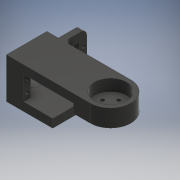
# Autodesk Inventor part: 第一臂-1
Saved by Autodesk Inventor 2017 (Build 210142000, 142)
## iProperties
Part Number: 第一臂-1
Material: 熱塑性塑膠樹脂
Document SubType Name: Modeling
Designer: Brian
Density: 1.28 g/cm^3
Appearance: 平滑 - 黑色
Mass: 49.9577 g
Surface Area: 163.253 cm^2
Volume: 39.0295 cm^3
Author: Brian
Autodesk Inventor part; units mm, degrees
ref_plane "YZ Plane" through (0, 0, 0) normal (1, 0, 0) x (0, 1, 0)
ref_plane "XZ Plane" through (0, 0, 0) normal (0, 1, 0) x (-1, 0, 0)
ref_plane "XY Plane" through (0, 0, 0) normal (0, 0, 1) x (1, 0, 0)
sketch "草圖1" plane through (0, 0, 0) normal (0, 0, 1) x (1, 0, 0)
  circle A0 centre (0, 0) radius 17.5
  circle A1 centre (120, 0) radius 17.5
  line L0 (0, 17.5) -> (120, 17.5)
  line L1 (120, 17.5) -> (120, -17.5)
  line L2 (120, -17.5) -> (0, -17.5)
  line L3 (0, -17.5) -> (0, 17.5)
  dimension "d0" = 35
  dimension "d1" = 35
  dimension "d4" = 120
  dimension "d5" = 35
  constraints: 8 end point, 3 coincident, 2 centre point, 2 midpoint, 2 parallel, 1 horizontal, 1 perpendicular
  measures "d0" diameter of A0
  measures "d1" diameter of A1
  measures "d4" distance of L0.start L0.end
  measures "d5" distance between parallel lines of L2 L0
extrude "擠出1" add sketch "草圖1" along normal blind 15
sketch "草圖2" plane through (0, 0, 15) normal (0, 0, 1) x (1, 0, 0)
  circle A0 centre (0, 0) radius 14
  arc A1 (120, -17.5) -> (120, 17.5) centre (120, 0) ccw projected
  circle A2 centre (120, 0) radius 14
  dimension "d6" = 28
  dimension "d7" = 28
  constraints: 2 centre point, 2 coincident
  measures "d6" diameter of A2
  measures "d7" diameter of A0
extrude "擠出2" cut sketch "草圖2" against normal blind 10
sketch "草圖5" plane through (0, 0, 0) normal (0, 0, -1) x (-1, 0, 0)
  circle A0 centre (0, 0) radius 14 projected
  line L0 (0, 17.5) -> (-120, 17.5) projected
  arc A1 (-120, 17.5) -> (-120, -17.5) centre (-120, 0) ccw projected
  line L1 (-120, -17.5) -> (0, -17.5) projected
  arc A2 (0, -17.5) -> (0, 17.5) centre (0, 0) ccw projected
  line L2 (0, 17.5) -> (-120, 17.5) projected
  line L3 (-87.5, 17.5) -> (-87.5, -17.5)
  line L4 (-120, -17.5) -> (0, -17.5) projected
  dimension "d13" = 50
  constraints: 2 end point, 2 point on line, 1 perpendicular
extrude "擠出4" add sketch "草圖5" along normal blind 20 contours A0 | A2 L1 L3 L0
ref_plane "工作平面1" through (0, 17.5, 11.7503) normal (0, 1, 0) x (1, 0, 0)
sketch "草圖6" plane through (0, 17.5, 11.7503) normal (0, 1, 0) x (1, 0, 0)
  line L0 (47.5, -10.5319) -> (-53.2917, -10.5319)
  line L1 (-53.2917, -10.5319) -> (-53.2917, 69.2461)
  line L2 (-53.2917, 69.2461) -> (47.5, 69.2461)
  line L3 (47.5, 69.2461) -> (47.5, -10.5319)
  line L4 (87.5, 11.7503) -> (87.5, 31.7503) projected
  point P0 (0, 11.7503)
  dimension "d19" = 40
  constraints: 8 end point, 2 parallel, 1 horizontal, 1 perpendicular
  measures "d19" distance between parallel lines of L4 L3
extrude "擠出5" cut sketch "草圖6" against normal through all
sketch "草圖7" plane through (120, 17.5, 15) normal (0, 1, 0) x (1, 0, 0)
  line L0 (-64.5, 7.25) -> (-14.5, 7.25)
  line L1 (-14.5, 7.25) -> (-14.5, 27.75)
  line L2 (-14.5, 27.75) -> (-64.5, 27.75)
  line L3 (-64.5, 27.75) -> (-64.5, 7.25)
  line L4 (0, 0) -> (-72.5, 0) projected
  line L5 (-72.5, 35) -> (-72.5, 0) projected
  point P0 (-120, 15)
  dimension "d20" = 20.5
  dimension "d21" = 7.25
  dimension "d22" = 8
  dimension "d23" = 50
  constraints: 8 end point, 2 parallel, 1 horizontal, 1 perpendicular
  measures "d20" distance of L2.end L0.start
  measures "d21" distance between parallel lines of L4 L0
  measures "d22" distance between parallel lines of L5 L3
  measures "d23" distance of L1.end L2.end
extrude "擠出6" cut sketch "草圖7" against normal through all
sketch "草圖8" plane through (47.5, -17.5, 15) normal (-1, 0, 0) x (0, 0, 1)
  line L0 (0, 0) -> (-35, 0) projected
  line L1 (0, 0) -> (-35, 35)
  line L2 (-35, 0) -> (-35, 35) projected
  circle A0 centre (-17.5, 17.5) radius 10.5
  point P0 (-15, 17.5)
  dimension "d26" = 21
  constraints: 2 end point, 1 centre point, 1 midpoint
  measures "d26" diameter of A0
extrude "擠出7" cut sketch "草圖8" against normal blind 10 contours A0 L1 | L1 A0
sketch "草圖9" plane through (120, 0, 5) normal (0, 0, 1) x (1, 0, 0)
  circle A0 centre (0, 0) radius 7
  circle A1 centre (0, 0) radius 14 projected
  line L0 (-7, 0) -> (0, 7)
  line L1 (0, 7) -> (7, 0)
  line L2 (7, 0) -> (0, -7)
  line L3 (0, -7) -> (-7, 0)
  point P0 (-120, 0)
  dimension "d29" = 14
  constraints: 8 end point, 1 coincident, 1 horizontal alignment, 12 other
hole "孔1" at (113, 0, 5) at (127, 0, 5) at (120, -7, 5) at (120, 7, 5) direction (0, 0, -1) diameter 3.2 depth 8 tip angle 118
sketch "草圖10" plane through (0, 0, 0) normal (0, 0, -1) x (-1, 0, 0)
  arc A0 (-120, 17.5) -> (-120, -17.5) centre (-120, 0) ccw projected
  circle A1 centre (-120, 0) radius 10
  circle A2 centre (-120, -7) radius 1.6 projected
  circle A3 centre (-113, 0) radius 1.6 projected
  circle A4 centre (-127, 0) radius 1.6 projected
  circle A5 centre (-120, 7) radius 1.6 projected
  line L0 (-105.5, -17.5) -> (-105.5, 17.5) projected
  line L1 (-105.5, 17.5) -> (-120, 17.5) projected
  arc A6 (-120, 17.5) -> (-120, -17.5) centre (-120, 0) ccw projected
  line L2 (-120, -17.5) -> (-105.5, -17.5) projected
  point P0 (0, 0)
  dimension "d37" = 20
  constraints: 1 centre point, 1 coincident
  measures "d37" diameter of A1
extrude "擠出8" add sketch "草圖10" along normal blind 0.2 contours A1
sketch "草圖13" plane through (55.5, -17.5, 7.75) normal (1, 0, 0) x (0, 0, -1)
  line L0 (20.5, 15.2224) -> (20.5, 0) projected
  line L1 (0, 15.2224) -> (0, 0) projected
  line L2 (20.5, 0) -> (0, 0)
  line L3 (0, 0) -> (0, 6)
  line L4 (0, 6) -> (20.5, 6)
  line L5 (20.5, 6) -> (20.5, 0)
  point P0 (7.75, 17.5)
  dimension "d46" = 6
  constraints: 8 end point, 2 parallel, 1 horizontal, 1 perpendicular, 1 point on line
  measures "d46" distance between parallel lines of L2 L4
extrude "擠出11" add sketch "草圖13" along normal blind 6.9
sketch "草圖14" plane through (120, 17.5, 15) normal (0, 1, 0) x (1, 0, 0)
  line L0 (-57.6, 7.25) -> (-64.5, 7.25) projected
  line L1 (0, 0) -> (-72.5, 0) projected
  line L2 (-57.6, 7.25) -> (-62.6, 7.25)
  line L3 (-62.6, 7.25) -> (-62.6, 0)
  line L4 (-62.6, 0) -> (-57.6, 0)
  line L5 (-57.6, 0) -> (-57.6, 7.25)
  line L6 (-57.6, 27.75) -> (-57.6, 7.25) projected
  line L7 (-72.5, 35) -> (-32.5, 35) projected
  line L8 (-57.6, 27.75) -> (-62.6, 27.75)
  line L9 (-62.6, 27.75) -> (-62.6, 35)
  line L10 (-62.6, 35) -> (-57.6, 35)
  line L11 (-57.6, 35) -> (-57.6, 27.75)
  point P0 (-120, 15)
  dimension "d49" = 5
  dimension "d50" = 5
  constraints: 16 end point, 4 parallel, 2 horizontal, 2 perpendicular, 2 point on line
  measures "d49" distance between parallel lines of L11 L9
  measures "d50" distance between parallel lines of L3 L5
extrude "擠出12" add sketch "草圖14" along normal blind 19.5
sketch "草圖15" plane through (57.4, 17.5, 7.75) normal (-1, 0, 0) x (0, 0, 1)
  line L0 (7.25, 19.5) -> (0, 19.5) projected
  line L1 (7.25, 19.5) -> (-27.75, 19.5)
  line L2 (-27.75, 19.5) -> (-27.75, 13)
  line L3 (-27.75, 13) -> (7.25, 13)
  line L4 (7.25, 13) -> (7.25, 19.5)
  point P0 (-7.75, -17.5)
  dimension "d53" = 35
  dimension "d54" = 6.5
  constraints: 8 end point, 2 parallel, 1 horizontal, 1 perpendicular
  measures "d53" distance of L0.start L1.end
  measures "d54" distance of L1.end L2.end
extrude "擠出13" add sketch "草圖15" against normal up to surface (5 mm away)
sketch "草圖16" plane through (62.4, -17.5, 7.75) normal (1, 0, 0) x (0, 0, -1)
  arc A0 (20.5, 19.7776) -> (0, 19.7776) centre (10.25, 17.5) ccw projected
  line L0 (5.25, 3.2) -> (15.25, 3.2)
  line L1 (15.25, 3.2) -> (15.25, 51.8)
  line L2 (15.25, 51.8) -> (5.25, 51.8)
  line L3 (5.25, 51.8) -> (5.25, 3.2)
  point P0 (7.75, 17.5)
  dimension "d57" = 5
  dimension "d58" = 10
  dimension "d59" = 34.3
  dimension "d60" = 48.6
  constraints: 8 end point, 2 parallel, 1 horizontal, 1 perpendicular
  measures "d57" distance from line of A0.centre L3
  measures "d58" distance of L1.end L2.end
  measures "d59" distance from line of A0.centre L2
  measures "d60" distance of L0.end L1.end
hole "孔2" at (62.4, -14.3, -7.5) at (62.4, -14.3, 2.5) at (62.4, 34.3, -7.5) at (62.4, 34.3, 2.5) direction (-1, 0, 0) diameter 3 depth 8 tip angle 118
fillet "圓角1" radius 5 2 edges at (59.9, 37, 15) (59.9, 37, -20)
fillet "圓角2" radius 5 2 edges at (62.4, 17.5, 11.375) (62.4, 17.5, -16.375)
